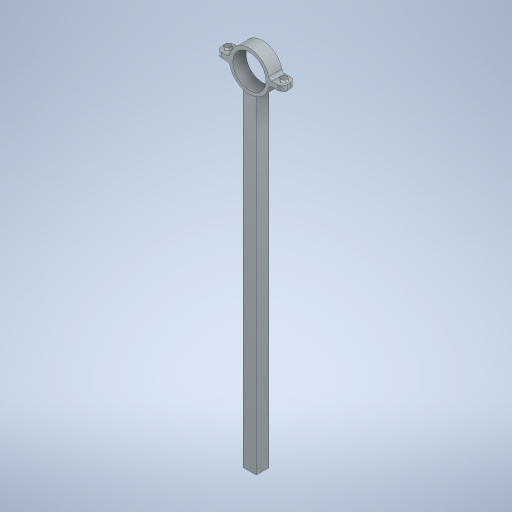
# Autodesk Inventor part: DN80-Rohrschelle-Staender
Saved by Autodesk Inventor 2023 (Build 270158000, 158)
## iProperties
Created: 2025-06-24
Part Number: DN80-Rohrschelle-Staender
Material: Generisch
Document SubType Name: Modeling
Designer: aurich
Density: 1 g/cm^3
Appearance: Vorgabe
Author: aurich
Autodesk Inventor part; units mm, degrees
ref_plane "YZ Plane" through (0, 0, 0) normal (1, 0, 0) x (0, 1, 0)
ref_plane "XY Plane" through (0, 0, 0) normal (0, 0, 1) x (1, 0, 0)
sketch "Skizze1" plane through (0, 0, 0) normal (0, 0, 1) x (1, 0, 0)
  circle A0 centre (0, 0) radius 50
  line L0 (100, 7.5) -> (100, -7.5)
  line L1 (-100, -7.5) -> (-100, 7.5)
  line L2 (-100, 7.5) -> (-68.374, 7.5)
  line L3 (68.374, 7.5) -> (100, 7.5)
  line L4 (100, -7.5) -> (68.374, -7.5)
  line L5 (-68.374, -7.5) -> (-100, -7.5)
  arc A1 (-58.6863, -15.0205) -> (58.6863, -15.0205) centre (0, 0) ccw
  arc A2 (58.6863, 15.0205) -> (-58.6863, 15.0205) centre (0, 0) ccw
  arc A3 (-68.374, 7.5) -> (-58.6863, 15.0205) centre (-68.374, 17.5) ccw
  arc A4 (-58.6863, -15.0205) -> (-68.374, -7.5) centre (-68.374, -17.5) ccw
  arc A5 (58.6863, 15.0205) -> (68.374, 7.5) centre (68.374, 17.5) ccw
  arc A6 (68.374, -7.5) -> (58.6863, -15.0205) centre (68.374, -17.5) ccw
  point P0 (-60.1119, 7.5)
  point P1 (60.1119, 7.5)
  point P2 (60.1119, -7.5)
  point P3 (-60.1119, -7.5)
  point P4 (-84.187, 7.5)
  point P5 (84.187, 7.5)
  point P6 (84.187, -7.5)
  point P7 (-84.187, -7.5)
  dimension "d1" = 100
  dimension "d4" = 100
  dimension "d5" = 100
  dimension "d6" = 10
  dimension "d7" = 7.5
  dimension "d8" = 7.5
  constraints: 16 point on circle, 12 end point, 8 tangent, 7 centre point, 5 parallel, 4 midpoint, 4 point on line, 3 equal radius, 2 coincident, 2 horizontal, 2 horizontal alignment, 2 perpendicular
  measures "d1" diameter of A0
  measures "d4" horizontal distance of point (0, 0) L1.end
  measures "d5" distance from line of point (0, 0) L0
  measures "d6" radius of A3
  measures "d7" distance from line of point (0, 0) L2
  measures "d8" vertical distance of point (0, 0) point (-84.187, -7.5)
extrude "Extrusion1" add sketch "Skizze1" along normal blind 40
fillet "Rundung1" radius 15 4 edges at (100, 0, 40) (100, 0, 0) (-100, 0, 40) (-100, 0, 0)
sketch "Skizze3" plane through (0, 0, 0) normal (0, 1, 0) x (-1, 0, 0)
  circle A0 centre (-85, 20) radius 10 construction
  line L0 (-85, 10) -> (-93.7649, 15.1858)
  line L1 (-93.7649, 24.8142) -> (-85, 30)
  line L2 (-85, 30) -> (-76.2351, 24.8142)
  line L3 (-76.2351, 24.8142) -> (-76.2351, 15.1858)
  line L4 (-85, 10) -> (-76.2351, 15.1858)
  line L5 (-93.7649, 24.8142) -> (-93.7649, 15.1858)
  arc A1 (-100, 15) -> (-85, 0) centre (-85, 15) ccw projected
  line L6 (-85, 0) -> (-68.374, 0) projected
  line L7 (-68.374, 0) -> (-68.374, 40) projected
  line L8 (-85, 40) -> (-68.374, 40) projected
  arc A2 (-85, 40) -> (-100, 25) centre (-85, 25) ccw projected
  line L9 (-100, 15) -> (-100, 25) projected
  arc A3 (85, 0) -> (100, 15) centre (85, 15) ccw projected
  line L10 (100, 15) -> (100, 25) projected
  arc A4 (100, 25) -> (85, 40) centre (85, 25) ccw projected
  line L11 (68.374, 40) -> (85, 40) projected
  line L12 (68.374, 0) -> (68.374, 40) projected
  line L13 (68.374, 0) -> (85, 0) projected
  line L14 (-85, 15) -> (-85, 25) construction
  line L15 (85, 15) -> (85, 25) construction
  circle A5 centre (85, 20) radius 10 construction
  line L16 (85, 10) -> (76.2351, 15.1858)
  line L17 (76.2351, 24.8142) -> (85, 30)
  line L18 (85, 30) -> (93.7649, 24.8142)
  line L19 (93.7649, 24.8142) -> (93.7649, 15.1858)
  line L20 (85, 10) -> (93.7649, 15.1858)
  line L21 (76.2351, 24.8142) -> (76.2351, 15.1858)
  line L22 (85, 15) -> (85, 25) construction
  point P0 (0, 0)
  point P1 (85, 20)
  dimension "d12" = 20
  dimension "d13" = 20
  constraints: 30 end point, 12 point on circle, 5 vertical, 4 horizontal alignment, 4 parallel, 3 midpoint, 2 centre point, 2 vertical alignment
  measures "d12" diameter of A0
  measures "d13" diameter of A5
extrude "Extrusion2" add sketch "Skizze3" along normal mid plane 30 contours L0 L5 L1 L2 L3 L4 | L16 L21 L17 L18 L19 L20
ref_plane "Arbeitsebene1" through (0, -52.25, 0) normal (0, 1, 0) x (-1, 0, 0)
sketch "Skizze4" plane through (0, -52.25, 0) normal (0, 1, 0) x (-1, 0, 0)
  line L0 (20, 39) -> (-20, 39)
  line L1 (-20, 39) -> (-20, 1)
  line L2 (-20, 1) -> (20, 1)
  line L3 (20, 1) -> (20, 39)
  point P0 (0, 0)
  dimension "d22" = 1
  dimension "d23" = 38
  dimension "d24" = 20
  dimension "d25" = 20
  constraints: 8 end point, 2 horizontal alignment, 2 vertical alignment
  measures "d22" distance from line of point (0, 0) L2
  measures "d23" distance between parallel lines of L0 L2
  measures "d24" distance from line of point (0, 0) L1
  measures "d25" distance from line of point (0, 0) L3
extrude "Extrusion3" add sketch "Skizze4" against normal blind 1000
